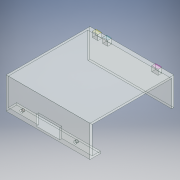
# Autodesk Inventor part: Top Plastic
Saved by Autodesk Inventor 2018 (Build 220112000, 112)
## iProperties
Created: 2018-02-19
Part Number: Top Plastic
Material: Generic
Document SubType Name: Modeling
Designer: Melda
Density: 1 g/cm^3
Appearance: Clear
Author: Melda
Autodesk Inventor part; units mm, degrees
ref_plane "YZ Plane" through (0, 0, 0) normal (1, 0, 0) x (0, 1, 0)
ref_plane "XZ Plane" through (0, 0, 0) normal (0, 1, 0) x (-1, 0, 0)
ref_plane "XY Plane" through (0, 0, 0) normal (0, 0, 1) x (1, 0, 0)
sketch "Sketch1" plane through (0, 0, 0) normal (1, 0, 0) x (0, 1, 0)
  line L0 (50.6514, 79.9086) -> (-9.3486, 79.9086)
  line L1 (-3.3486, -80.0914) -> (50.6514, -80.0914)
  line L2 (50.6514, -80.0914) -> (50.6514, 79.9086)
  line L3 (-9.3486, 79.9086) -> (-9.3486, 59.9086)
  line L4 (-9.3486, 59.9086) -> (-5.3486, 59.9086)
  line L5 (-5.3486, 59.9086) -> (-5.3486, 75.9086)
  line L6 (-5.3486, 75.9086) -> (46.6514, 75.9086)
  line L7 (46.6514, 75.9086) -> (46.6514, -76.0914)
  line L8 (46.6514, -76.0914) -> (-3.3486, -76.0914)
  line L9 (-3.3486, -76.0914) -> (-3.3486, -80.0914)
  point P0 (0, 0)
  dimension "d0" = 160
  dimension "d1" = 54
  dimension "d2" = 60
  dimension "d3" = 20
  dimension "d4" = 4
  dimension "d5" = 4
  dimension "d6" = 4
  dimension "d7" = 4
  dimension "d8" = 4
  dimension "d9" = 4
  constraints: 20 end point, 5 perpendicular, 2 horizontal, 1 parallel, 1 vertical
  measures "d0" distance of L1.end L0.start
  measures "d1" distance of L1.start L1.end
  measures "d2" distance of L0.start L0.end
  measures "d3" distance of L0.end L3.end
  measures "d4" distance of L3.end L4.end
  measures "d5" distance from line of L0 L5.end
  measures "d6" distance from line of L0 L6.end
  measures "d7" distance from line of L2 L6.end
  measures "d8" distance from line of L1 L7.end
  measures "d9" distance of L8.end L1.start
extrude "Extrusion1" add sketch "Sketch1" along normal blind 160
sketch "Sketch2" plane through (0, -9.3486, 79.9086) normal (0, 0, 1) x (1, 0, 0)
  line L0 (57.5, 4) -> (102.5, 4)
  line L1 (102.5, 4) -> (102.5, 24)
  line L2 (102.5, 24) -> (57.5, 24)
  line L3 (57.5, 24) -> (57.5, 4)
  line L4 (57.5, 4) -> (102.5, 24) construction
  line L5 (102.5, 4) -> (57.5, 24) construction
  line L6 (0, 0) -> (160, 0) projected
  line L7 (160, 60) -> (160, 0) projected
  point P0 (0, 9.3486)
  point P1 (80, 14)
  dimension "d12" = 45
  dimension "d13" = 4
  dimension "d14" = 20
  dimension "d15" = 80
  constraints: 12 end point, 2 midpoint, 2 parallel, 1 horizontal, 1 perpendicular
  measures "d12" distance of L1.end L2.end
  measures "d13" distance between parallel lines of L6 L0
  measures "d14" distance of L0.end L1.end
  measures "d15" distance from line of L7 point (80, 14)
extrude "Extrusion2" cut sketch "Sketch2" against normal blind 5
sketch "Sketch3" plane through (0, -9.3486, 79.9086) normal (0, 0, 1) x (1, 0, 0)
  circle A0 centre (28.75, 14) radius 2.5
  circle A1 centre (131.25, 14) radius 2.5
  line L0 (0, 60) -> (0, 0) projected
  line L1 (57.5, 4) -> (57.5, 24) projected
  line L2 (160, 60) -> (160, 0) projected
  line L3 (102.5, 4) -> (57.5, 4) projected
  line L4 (57.5, 24) -> (102.5, 24) projected
  line L5 (0, 0) -> (160, 0) projected
  circle A2 centre (28.75, 14) radius 2.75
  circle A3 centre (131.25, 14) radius 2.75
  point P0 (0, 9.3486)
  dimension "d18" = 5
  dimension "d19" = 57.5
  dimension "d20" = 28.75
  dimension "d21" = 28.75
  dimension "d22" = 20
  dimension "d23" = 14
  dimension "d24" = 4
  dimension "d25" = 14
  dimension "d26" = 5.5
  constraints: 4 centre point, 2 coincident, 2 equal radius
  measures "d18" diameter of A0
  measures "d19" distance between parallel lines of L0 L1
  measures "d20" distance from line of L0 A0.centre
  measures "d21" distance from line of L2 A1.centre
  measures "d22" distance between parallel lines of L3 L4
  measures "d23" distance from line of L5 A1.centre
  measures "d24" distance between parallel lines of L5 L3
  measures "d25" distance from line of L5 A0.centre
  measures "d26" diameter of A2
extrude "Extrusion3" cut sketch "Sketch3" against normal blind 5
fillet "Fillet1" radius 2 2 edges at (26.25, 4.6514, 79.9086) (128.75, 4.6514, 79.9086)
sketch "Sketch4" plane through (0, 50.6514, 79.9086) normal (0, 1, 0) x (1, 0, 0)
  line L0 (20.0495, 144.1884) -> (30.8697, 144.1884)
  line L1 (30.8697, 144.1884) -> (30.8697, 151.4018)
  line L2 (30.8697, 151.4018) -> (20.0495, 151.4018)
  line L3 (20.0495, 151.4018) -> (20.0495, 144.1884)
  line L4 (39.8865, 144.1884) -> (49.805, 144.1884)
  line L5 (49.805, 144.1884) -> (49.805, 151.4018)
  line L6 (49.805, 151.4018) -> (39.8865, 151.4018)
  line L7 (39.8865, 151.4018) -> (39.8865, 144.1884)
  line L8 (133.6613, 144.1884) -> (145.6838, 144.1884)
  line L9 (145.6838, 144.1884) -> (145.6838, 151.4018)
  line L10 (145.6838, 151.4018) -> (133.6613, 151.4018)
  line L11 (133.6613, 151.4018) -> (133.6613, 144.1884)
  point P0 (0, 79.9086)
  constraints: 24 end point, 6 parallel, 4 point on line, 3 horizontal, 3 perpendicular
extrude "Extrusion4" add sketch "Sketch4" along normal blind 10
body "Solid1"
